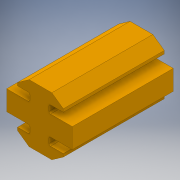
# Autodesk Inventor part: 20X20Connector
Saved by Autodesk Inventor 2017 (Build 210142000, 142)
## iProperties
Created: 2018-01-13
Part Number: 20X20Connector
Material: Generic
Document SubType Name: Modeling
Designer: User
Density: 1 g/cm^3
Appearance: Default(1)
Author: User
Autodesk Inventor part; units mm, degrees
ref_plane "YZ Plane" through (0, 0, 0) normal (1, 0, 0) x (0, 1, 0)
ref_plane "XZ Plane" through (0, 0, 0) normal (0, 1, 0) x (-1, 0, 0)
ref_plane "XY Plane" through (0, 0, 0) normal (0, 0, 1) x (1, 0, 0)
sketch "Sketch1" plane through (0, 0, 0) normal (0, 0, 1) x (1, 0, 0)
  line L0 (-8.7854, 4.1412) -> (7.7246, 4.1412)
  line L1 (7.7246, 1.6412) -> (1.8496, 1.6412)
  line L2 (1.8496, 1.6412) -> (1.8496, -0.3588)
  line L3 (1.8496, -0.3588) -> (5.4596, -0.3588)
  line L4 (2.5721, -3.1588) -> (-3.1429, -3.1588)
  line L5 (-3.1429, -3.1588) -> (-6.0304, -1.1208)
  line L6 (-6.0304, -1.1208) -> (-6.0304, -0.3588)
  line L7 (-6.0304, -0.3588) -> (-2.9104, -0.3588)
  line L8 (-2.9104, -0.3588) -> (-2.9104, 1.6412)
  line L9 (-2.9104, 1.6412) -> (-8.7854, 1.6412)
  line L10 (-8.7854, 1.6412) -> (-8.7854, 4.1412)
  line L11 (5.4596, -0.3588) -> (5.4596, -1.1208)
  line L12 (5.4596, -1.1208) -> (2.5721, -3.1588)
  line L13 (7.7246, 4.1412) -> (7.7246, 1.6412)
  point P0 (0, 0)
  dimension "d0" = 2.5
  dimension "d1" = 2
  dimension "d2" = 4.76
  dimension "d3" = 11.49
  dimension "d4" = 2.755
  dimension "d5" = 5.715
  dimension "d6" = 5.6425
  dimension "d7" = 5.875
  dimension "d8" = 0.762
  dimension "d9" = 0.762
  dimension "d11" = 144.786
  dimension "d12" = 2.8875
  dimension "d14" = 16.51
  constraints: 28 end point, 5 perpendicular, 4 point on line, 1 horizontal, 1 vertical
  measures "d0" distance between parallel lines of L9 L0
  measures "d1" distance between parallel lines of L7 L9
  measures "d2" distance between parallel lines of L2 L8
  measures "d3" distance between parallel lines of L6 L11
  measures "d4" distance between parallel lines of L6 L10
  measures "d5" distance of L4.start L4.end
  measures "d6" distance from line of L4.end L10
  measures "d7" distance between parallel lines of L10 L8
  measures "d8" distance of L5.end L6.end
  measures "d9" distance of L3.end L11.end
  measures "d11" angle of L12 L4
  measures "d12" distance from line of L4.start L11
  measures "d14" distance between parallel lines of L13 L10
extrude "Extrusion1" add sketch "Sketch1" along normal blind 25.4
ref_plane "Work Plane1" through (-8.7854, 4.1412, 0) normal (0, 1, 0) x (1, 0, 0)
fillet "Fillet2" radius 0.3969 4 edges at (1.8496, -0.3588, 12.7) (1.8496, 1.6412, 12.7) (-2.9104, 1.6412, 12.7) (-2.9104, -0.3588, 12.7)
mirror "Mirror2" about plane through (-8.7854, 4.1412, 0) normal (0, 1, 0) of "Fillet2", "Extrusion1"
equation "\"d4\" = -0.5 * d3 + 0.5 * d13"
equation "\"d6\" = -0.5 * d5 + 0.5 * d13"
equation "\"d7\" = -0.5 * d2 + 0.5 * d14"
equation "\"d9\" = d8"
equation "\"d13\" = 17"
body "Solid1"
